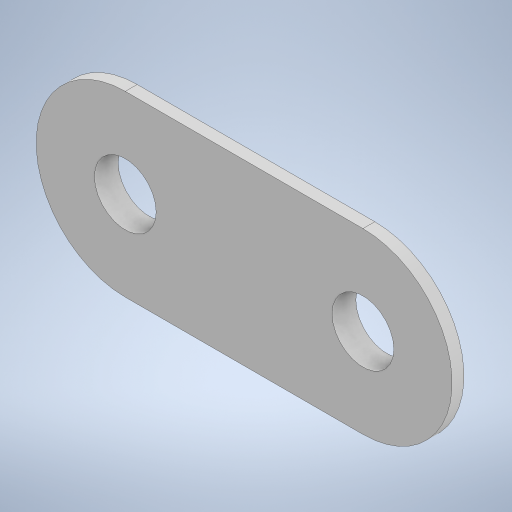
# Autodesk Inventor part: Belt Holder
Saved by Autodesk Inventor 2023.1 (Build 271208000, 208)
## iProperties
Created: 2022-10-29
Part Number: Belt Holder
Material: Generic
Document SubType Name: Modeling
Designer: nicol
Density: 1 g/cm^3
Appearance: Default
Author: nicol
Autodesk Inventor part; units mm, degrees
ref_plane "YZ Plane" through (0, 0, 0) normal (1, 0, 0) x (0, 1, 0)
ref_plane "XZ Plane" through (0, 0, 0) normal (0, 1, 0) x (-1, 0, 0)
ref_plane "XY Plane" through (0, 0, 0) normal (0, 0, 1) x (1, 0, 0)
sketch "Sketch1" plane through (0, 0, 0) normal (0, 0, 1) x (1, 0, 0)
  circle A0 centre (0, 0) radius 7.5
  circle A1 centre (20, 0) radius 7.5
  line L0 (0, 7.5) -> (20, 7.5)
  line L1 (0, -7.5) -> (20, -7.5)
  circle A2 centre (0, 0) radius 3.2
  circle A3 centre (20, 0) radius 3.2
  circle A4 centre (20, 0) radius 2.6
  circle A5 centre (0, 0) radius 2.6
  dimension "d0" = 20
  dimension "d1" = 15
  dimension "d6" = 5.2
  dimension "d7" = 5.2
  dimension "d10" = 0.6
  dimension "d11" = 0.6
  constraints: 6 centre point, 5 coincident, 4 end point, 4 point on circle, 4 tangent, 1 equal radius, 1 horizontal
  measures "d0" distance of A1.centre point (0, 0)
  measures "d1" diameter of A0
  measures "d6" diameter of A4
  measures "d7" diameter of A5
  measures "d10" radial gap between concentric circles of A3 A4
  measures "d11" radial gap between concentric circles of A2 A5
extrude "Extrusion1" add sketch "Sketch1" along normal blind 1 contours A0 | A0 L0 A1 L1 | A1 | A2 | A3
extrude "Extrusion2" add sketch "Sketch1" against normal blind 1 contours A2 | A3
equation "\"d6\" = d7"
equation "\"d11\" = d10"
body "Solid1"
